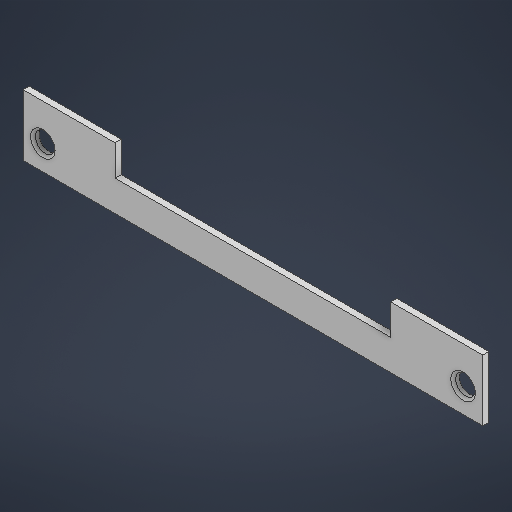
# Autodesk Inventor part: oslonka
Saved by Autodesk Inventor 2026.1 (Build 301233020, 233B)
## iProperties
Created: 2025-11-22
Part Number: oslonka
Material: Generic
Document SubType Name: Modeling
Designer: Jan
Density: 1 g/cm^3
Appearance: Default
Author: Jan
Autodesk Inventor part; units mm, degrees
ref_plane "YZ Plane" through (0, 0, 0) normal (1, 0, 0) x (0, 1, 0)
ref_plane "XZ Plane" through (0, 0, 0) normal (0, 1, 0) x (-1, 0, 0)
ref_plane "XY Plane" through (0, 0, 0) normal (0, 0, 1) x (1, 0, 0)
sketch "Sketch1" plane through (0, 0, 0) normal (0, 0, 1) x (1, 0, 0)
  line L0 (0, 0) -> (75, 0)
  line L1 (75, 0) -> (75, 10)
  line L2 (75, 10) -> (0, 10)
  line L3 (0, 10) -> (0, 0)
  line L4 (15, 10) -> (15, 5)
  line L5 (15, 5) -> (60, 5)
  line L6 (60, 5) -> (60, 10)
  circle A0 centre (3.2, 4) radius 1.6
  line L7 (37.5, 10) -> (37.5, 6.6559) construction
  circle A1 centre (71.8, 4) radius 1.6
  point P0 (0, 5)
  dimension "d0" = 75
  dimension "d1" = 10
  dimension "d3" = 5
  dimension "d4" = 45
  dimension "d5" = 3.2
  dimension "d7" = 4
  dimension "d10" = 3.2
  constraints: 16 end point, 3 perpendicular, 2 centre point, 2 midpoint, 2 parallel, 2 point on line, 2 vertical, 1 horizontal, 1 symmetric about line, 1 other
  measures "d0" distance of L2.end L1.end
  measures "d1" distance of L1.end L0.end
  measures "d3" distance of L4.start L4.end
  measures "d4" distance of L4.end L5.end
  measures "d5" diameter of A0
  measures "d7" distance from line of L0 A0.centre
  measures "d10" distance from line of L3 A0.centre
extrude "Extrusion1" add sketch "Sketch1" along normal blind 1 contours L3 L2 L4 L5 L6 L1 L0
chamfer "Chamfer1" distance 0.4 angle 45 2 edges at (1.6, 4, 1) (70.2, 4, 1)
body "Solid1"
